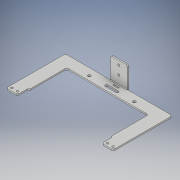
# Autodesk Inventor part: Battery Mount C Plate
Saved by Autodesk Inventor 2017.3 (Build 213256000, 256)
## iProperties
Created: 2019-01-21
Part Number: Battery Mount C Plate
Material: Generic
Document SubType Name: Modeling
Designer: jb0839
Density: 1 g/cm^3
Appearance: Default
Author: jb0839
Autodesk Inventor part; units mm, degrees
ref_plane "YZ Plane" through (0, 0, 0) normal (1, 0, 0) x (0, 1, 0)
ref_plane "XZ Plane" through (0, 0, 0) normal (0, 1, 0) x (-1, 0, 0)
ref_plane "XY Plane" through (0, 0, 0) normal (0, 0, 1) x (1, 0, 0)
sketch "Sketch1" plane through (0, 0, 0) normal (0, 0, 1) x (1, 0, 0)
  line L0 (0, 0) -> (133.35, 0)
  line L1 (133.35, 0) -> (133.35, 241.3)
  line L2 (133.35, 241.3) -> (0, 241.3)
  line L3 (0, 241.3) -> (0, 0)
  line L4 (133.35, 0) -> (133.35, 25.4)
  line L5 (133.35, 0) -> (158.75, 0) construction
  line L6 (133.35, 25.4) -> (111.125, 25.4)
  line L7 (133.35, 25.4) -> (155.575, 25.4) construction
  line L8 (107.95, 28.575) -> (111.125, 25.4)
  line L9 (107.95, 28.575) -> (25.4, 28.575)
  line L10 (133.35, 25.4) -> (111.125, 25.4)
  line L11 (107.95, 28.575) -> (111.125, 25.4)
  line L12 (107.95, 28.575) -> (25.4, 28.575)
  line L13 (0, 120.65) -> (133.35, 120.65)
  line L14 (25.4, 28.575) -> (25.4, 120.65)
  line L15 (133.35, 25.4) -> (127, 25.4)
  line L16 (127, 25.4) -> (127, 19.05)
  line L17 (127, 19.05) -> (127, 6.35)
  line L18 (107.95, 212.725) -> (111.125, 215.9)
  line L19 (107.95, 212.725) -> (25.4, 212.725)
  line L20 (133.35, 215.9) -> (111.125, 215.9)
  line L21 (25.4, 212.725) -> (25.4, 120.65)
  line L22 (25.4, 120.65) -> (25.4, 212.725)
  line L23 (25.4, 212.725) -> (107.95, 212.725)
  line L24 (107.95, 212.725) -> (111.125, 215.9)
  line L25 (111.125, 215.9) -> (133.35, 215.9)
  line L26 (133.35, 215.9) -> (133.35, 241.3)
  line L27 (133.35, 241.3) -> (0, 241.3)
  line L28 (0, 241.3) -> (0, 120.65)
  point P0 (127, 234.95)
  point P1 (127, 222.25)
  dimension "d0" = 133.35
  dimension "d1" = 241.3
  dimension "d2" = 25.4
  dimension "d3" = 90
  dimension "d5" = 22.225
  dimension "d6" = 180
  dimension "d9" = 6.35
  dimension "d10" = 6.35
  dimension "d11" = 12.7
  constraints: 58 end point, 7 collinear, 7 perpendicular, 6 symmetric about line, 4 horizontal, 3 point on line, 2 coincident, 2 equal length, 2 midpoint, 2 parallel
  measures "d0" distance of L2.end L1.end
  measures "d1" distance of L1.end L0.end
  measures "d2" distance of L0.end L4.end
  measures "d3" angle of L5 L4
  measures "d5" distance of L4.end L6.end
  measures "d6" angle of L6 L7
  measures "d9" distance of L4.end L15.end
  measures "d10" distance of L15.end L16.end
  measures "d11" distance of L16.end L17.end
extrude "Extrusion1" add sketch "Sketch1" along normal blind 3.175 contours L3 L13 L14 L9 L8 L6 L1 L0 | L3 L2 L1 L20 L18 L19 L21 L13
chamfer "Chamfer1" distance 3.175 angle 45 6 edges at (133.35, 241.3, 1.5875) (133.35, 215.9, 1.5875) (0, 241.3, 1.5875) (0, 0, 1.5875) (133.35, 0, 1.5875) (133.35, 25.4, 1.5875)
hole "Hole1" at (127, 6.35, 0) at (127, 19.05, 0) at (127, 222.25, 0) at (127, 234.95, 0) direction (0, 0, 1) diameter 4.7625 end through all
sketch "Sketch2" plane through (0, 0, 3.175) normal (0, 0, 1) x (1, 0, 0)
  line L0 (25.4, 28.575) -> (25.4, 212.725) projected
  line L1 (25.4, 120.65) -> (0, 120.65)
  line L2 (25.4, 120.65) -> (15.875, 120.65)
  line L3 (25.4, 120.65) -> (34.925, 120.65) construction
  line L4 (15.875, 120.65) -> (19.05, 120.65)
  line L5 (19.05, 120.65) -> (12.7, 120.65)
  line L6 (12.7, 120.65) -> (19.05, 120.65)
  line L7 (19.05, 120.65) -> (19.05, 135.7313)
  line L8 (19.05, 135.7313) -> (12.7, 135.7313)
  line L9 (12.7, 135.7313) -> (12.7, 120.65)
  line L10 (12.7, 135.7313) -> (19.05, 135.7313)
  line L11 (19.05, 135.7313) -> (19.05, 105.5688)
  line L12 (19.05, 105.5688) -> (12.7, 105.5688)
  line L13 (12.7, 105.5688) -> (12.7, 135.7313)
  line L14 (0, 120.65) -> (6.35, 120.65)
  line L15 (0, 120.65) -> (6.35, 120.65) construction
  line L16 (6.35, 120.65) -> (4.7625, 120.65)
  line L17 (4.7625, 120.65) -> (7.9375, 120.65)
  line L18 (7.9375, 120.65) -> (4.7625, 120.65)
  line L19 (4.7625, 120.65) -> (4.7625, 127)
  line L20 (4.7625, 127) -> (7.9375, 127)
  line L21 (7.9375, 127) -> (7.9375, 120.65)
  line L22 (4.7625, 127) -> (7.9375, 127)
  line L23 (7.9375, 127) -> (7.9375, 114.3)
  line L24 (7.9375, 114.3) -> (4.7625, 114.3)
  line L25 (4.7625, 114.3) -> (4.7625, 127)
  line L26 (25.4, 120.65) -> (19.05, 120.65)
  line L27 (15.875, 120.65) -> (15.875, 171.45)
  line L28 (15.875, 120.65) -> (66.675, 120.65) construction
  line L29 (15.875, 171.45) -> (15.875, 69.85)
  point P0 (0, 0)
  point P1 (15.875, 69.85)
  point P2 (15.875, 171.45)
  dimension "d24" = 9.525
  dimension "d25" = 180
  dimension "d26" = 3.175
  dimension "d27" = 0
  dimension "d28" = 6.35
  dimension "d29" = 0
  dimension "d30" = 6.35
  dimension "d31" = 15.0813
  dimension "d32" = 6.35
  dimension "d33" = 30.1625
  dimension "d34" = 6.35
  dimension "d35" = 0
  dimension "d36" = 1.5875
  dimension "d37" = 0
  dimension "d38" = 3.175
  dimension "d39" = 0
  dimension "d40" = 3.175
  dimension "d41" = 6.35
  dimension "d42" = 3.175
  dimension "d43" = 12.7
  dimension "d44" = 6.35
  dimension "d58" = 50.8
  dimension "d59" = 90
  dimension "d60" = 101.6
  dimension "d61" = 0
  constraints: 58 end point, 9 horizontal, 8 parallel, 7 collinear, 5 perpendicular, 3 equal length, 1 midpoint
  measures "d24" distance of L1.start L2.end
  measures "d25" angle of L2 L3
  measures "d26" distance of L2.end L4.end
  measures "d27" distance between parallel lines of L4 L2
  measures "d28" distance of L4.end L5.end
  measures "d29" distance between parallel lines of L5 L4
  measures "d30" distance of L8.end L7.end
  measures "d31" distance of L7.end L6.end
  measures "d32" distance of L11.end L12.end
  measures "d33" distance of L10.end L11.end
  measures "d34" distance of L1.end L14.end
  measures "d35" distance between parallel lines of L14 L15
  measures "d36" distance of L14.end L16.end
  measures "d37" distance between parallel lines of L16 L14
  measures "d38" distance of L16.end L17.end
  measures "d39" distance between parallel lines of L17 L16
  measures "d40" distance of L19.end L20.end
  measures "d41" distance of L18.end L19.end
  measures "d42" distance of L23.end L24.end
  measures "d43" distance of L22.end L23.end
  measures "d44" distance of L1.start L6.end
  measures "d58" distance of L2.end L27.end
  measures "d59" angle of L28 L27
  measures "d60" distance of L27.end L29.end
  measures "d61" distance between parallel lines of L29 L27
extrude "Extrusion2" cut sketch "Sketch2" against normal blind 3.175
hole "Hole2" at (15.875, 69.85, 3.175) at (15.875, 171.45, 3.175) direction (0, 0, -1) diameter 6.35 end through all
fillet "Fillet1" radius 3.175 4 edges at (12.7, 135.7313, 1.5875) (19.05, 135.7313, 1.5875) (12.7, 105.5688, 1.5875) (19.05, 105.5688, 1.5875)
fillet "Fillet2" radius 1.5875 4 edges at (4.7625, 114.3, 1.5875) (7.9375, 114.3, 1.5875) (4.7625, 127, 1.5875) (7.9375, 127, 1.5875)
sketch "Sketch3" plane through (0, 0, 3.175) normal (0, 0, 1) x (1, 0, 0)
  line L0 (4.7625, 115.8875) -> (4.7625, 125.4125) projected
  line L1 (4.7625, 120.65) -> (0, 120.65)
  line L2 (0, 238.125) -> (0, 3.175) projected
  line L3 (0, 120.65) -> (-3.175, 120.65)
  line L4 (-3.175, 120.65) -> (-3.175, 139.7)
  line L5 (-3.175, 139.7) -> (0, 139.7)
  line L6 (0, 139.7) -> (0, 120.65)
  line L7 (-3.175, 139.7) -> (0, 139.7)
  line L8 (0, 139.7) -> (0, 101.6)
  line L9 (0, 101.6) -> (-3.175, 101.6)
  line L10 (-3.175, 101.6) -> (-3.175, 139.7)
  point P0 (0, 0)
  dimension "d64" = 3.175
  dimension "d65" = 19.05
  dimension "d66" = 3.175
  dimension "d67" = 38.1
  constraints: 18 end point, 4 parallel, 2 horizontal, 2 midpoint, 2 perpendicular
  measures "d64" distance of L4.end L5.end
  measures "d65" distance of L3.end L4.end
  measures "d66" distance of L8.end L9.end
  measures "d67" distance of L7.end L8.end
extrude "Extrusion3" add sketch "Sketch3" along normal blind 47.625 and the other way blind 3.175
fillet "Fillet3" radius 1.5875 1 edges at (0, 120.65, 3.175)
fillet "Fillet4" radius 3.175 1 edges at (-3.175, 120.65, 0)
chamfer "Chamfer2" distance 3.175 angle 45 4 edges at (25.4, 28.575, 1.5875) (25.4, 212.725, 1.5875) (-1.5875, 101.6, 50.8) (-1.5875, 139.7, 50.8)
sketch "Sketch4" plane through (0, 101.6, 4.7625) normal (1, 0, 0) x (0, 0, -1)
  line L0 (-46.0375, 3.175) -> (-46.0375, 34.925) projected
  line L1 (-46.0375, 19.05) -> (-36.5125, 19.05)
  line L2 (-46.0375, 19.05) -> (-36.5125, 19.05) construction
  line L3 (-46.0375, 19.05) -> (-17.4625, 19.05)
  line L4 (-46.0375, 19.05) -> (-17.4625, 19.05) construction
  point P0 (4.7625, -101.6)
  dimension "d77" = 9.525
  dimension "d78" = 0
  dimension "d79" = 28.575
  dimension "d80" = 0
  constraints: 8 end point, 3 collinear, 3 horizontal, 2 coincident, 1 midpoint
  measures "d77" distance of L1.start L1.end
  measures "d78" distance between parallel lines of L1 L2
  measures "d79" distance of L1.start L3.end
  measures "d80" distance between parallel lines of L3 L4
hole "Hole3" at (0, 120.65, 41.275) at (0, 120.65, 22.225) direction (-1, 0, 0) diameter 4.7625 end through all
ref_plane "Work Plane1" through (3.175, 120.65, 0) normal (0, 1, 0) x (1, 0, 0)
ref_plane "Work Plane2" through (127, 3.175, 0) normal (1, 0, 0) x (0, 0, -1)
body "Solid1"
